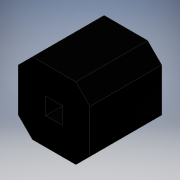
# Autodesk Inventor part: Pin Stopper 0.6mm
Saved by Autodesk Inventor 2016 (Build 200138000, 138)
## iProperties
Created: 2016-01-25
Part Number: Pin Stopper 0.6mm
Material: PAEK Plastic
Document SubType Name: Modeling
Designer: larraguetajunior
Density: 1.32 g/cm^3
Appearance: Smooth - White
Mass: 0.0187475 g
Surface Area: 0.401098 cm^2
Volume: 0.0142027 cm^3
Author: larraguetajunior
Autodesk Inventor part; units mm, degrees
ref_plane "YZ Plane" through (0, 0, 0) normal (1, 0, 0) x (0, 1, 0)
ref_plane "XZ Plane" through (0, 0, 0) normal (0, 1, 0) x (-1, 0, 0)
ref_plane "XY Plane" through (0, 0, 0) normal (0, 0, 1) x (1, 0, 0)
sketch "Sketch1" plane through (0, 0, 0) normal (0, 1, 0) x (-1, 0, 0)
  line L0 (1.27, 1.27) -> (-1.27, 1.27)
  line L1 (-1.27, 1.27) -> (-1.27, -1.27)
  line L2 (-1.27, -1.27) -> (1.27, -1.27)
  line L3 (1.27, -1.27) -> (1.27, 1.27)
  line L4 (1.27, 1.27) -> (-1.27, -1.27) construction
  line L5 (-1.27, 1.27) -> (1.27, -1.27) construction
  line L6 (0.3, -0.3) -> (-0.3, -0.3)
  line L7 (-0.3, -0.3) -> (-0.3, 0.3)
  line L8 (-0.3, 0.3) -> (0.3, 0.3)
  line L9 (0.3, 0.3) -> (0.3, -0.3)
  line L10 (0.3, -0.3) -> (-0.3, 0.3) construction
  line L11 (-0.3, -0.3) -> (0.3, 0.3) construction
  point P0 (0, 0)
  dimension "d0" = 2.54
  dimension "d1" = 2.54
  dimension "d7" = 0.6
  dimension "d8" = 0.6
  constraints: 24 end point, 4 midpoint, 4 parallel, 2 horizontal, 2 perpendicular
  measures "d0" distance of L2.end L1.end
  measures "d1" distance of L1.end L0.end
  measures "d7" distance of L7.end L8.end
  measures "d8" distance of L6.end L7.end
extrude "Extrusion1" add sketch "Sketch1" along normal mid plane 2.54
chamfer "Chamfer1" distance 0.5 angle 45 4 edges at (1.27, 0, 1.27) (1.27, 0, -1.27) (-1.27, 0, -1.27) (-1.27, 0, 1.27)
body "Solid1"
